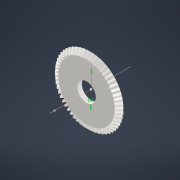
# Autodesk Inventor part: Bevel Gear1
Saved by Autodesk Inventor 2022 (Build 260153000, 153)
## iProperties
CustomPartVersion: 1
Created: 2021-09-10
Part Number: Bevel Gear1
Material: Steel, Mild
Document SubType Name: Modeling
Designer: Andres
Categories: <?xml version="1.0" encoding="UTF-16"?> <MemberInstance><Categories><FamilyTemplate><FamilyTemplateParameter ValueType="xs:double" Id="1" ObjectReferenceKey="da_z" ObjectType="kUserParameterObject"/><FamilyTemplateParameter ValueType="xs:double" Id="2" ObjectReferenceKey="da_b" ObjectType="kUserParameterObject"/><FamilyTemplateParameter ValueType="xs:double" Id="3" ObjectReferenceKey="da_beta" ObjectType="kUserParameterObject"/><FamilyTemplateParameter ValueType="xs:double" Id="4" ObjectReferenceKey="da_dae" ObjectType="kUserParameterObject"/><FamilyTemplateParameter ValueType="xs:double" Id="5" ObjectReferenceKey="da_ve" ObjectType="kUserParameterObject"/><FamilyTemplateParameter ValueType="xs:double" Id="6" ObjectReferenceKey="da_omega" ObjectType="kUserParameterObject"/><FamilyTemplateParameter ValueType="xs:string" Id="7" ObjectReferenceKey="EAIAABAAAAAAHwAAAAAAAIAAAAAAAAAA" ObjectType="83914240" SubObjectId="SurfaceGeometry"/></FamilyTemplate><ParamToTemplateMap><ParamToTemplate CategoryParameter="//CategoryParameter[@InternalName='046C89C9-8512-4d59-83FE-43B91F4F132A']" TemplateParameter="1"/><ParamToTemplate CategoryParameter="//CategoryParameter[@InternalName='2552DF32-E462-4b46-AEBF-C6C7768E72AC']" TemplateParameter="2"/><ParamToTemplate CategoryParameter="//CategoryParameter[@InternalName='C9EE641D-15FC-4fae-A226-E94C4372FDD7']" TemplateParameter="3"/><ParamToTemplate><ParamToTemplate CategoryParameter="//CategoryParameter[@InternalName='00B6519A-459B-49c7-AD84-2E56D39A5744']" ConstantValue="0.000000"/></ParamToTemplate><ParamToTemplate><ParamToTemplate CategoryParameter="//CategoryParameter[@InternalName='04B31F0E-C7A6-4894-AA32-9629BEFACF47']" ConstantValue="1.000000"/></ParamToTemplate><ParamToTemplate><ParamToTemplate CategoryParameter="//CategoryParameter[@InternalName='43CBEC2E-7847-49e7-A936-2F7889FCB2D9']" ConstantValue="0.200000"/></ParamToTemplate><ParamToTemplate><ParamToTemplate CategoryParameter="//CategoryParameter[@InternalName='B1EFC894-105D-4ebd-86BF-FA20ED196853']" ConstantValue="0.300000"/></ParamToTemplate><ParamToTemplate><ParamToTemplate CategoryParameter="//CategoryParameter[@InternalName='51175063-3D10-4879-93E8-6246FE8B403D']" ConstantValue="2060000000.000000"/></ParamToTemplate><ParamToTemplate><ParamToTemplate CategoryParameter="//CategoryParameter[@InternalName='A3A52E27-4454-46a9-B0BD-C932399B70AF']" ConstantValue="0.300000"/></ParamToTemplate><ParamToTemplate CategoryParameter="//CategoryParameter[@InternalName='2A200944-5A8C-41ca-B96E-8520D2E510F1']" TemplateParameter="4"/><ParamToTemplate><ParamToTemplate CategoryParameter="//CategoryParameter[@InternalName='1A637F62-92C8-44bc-B81F-10802510B579']" ConstantValue="9.677909"/></ParamToTemplate><ParamToTemplate CategoryParameter="//CategoryParameter[@InternalName='B52DD4BE-6863-48fb-BF58-89EF6F9EC65C']" TemplateParameter="5"/><ParamToTemplate><ParamToTemplate CategoryParameter="//CategoryParameter[@InternalName='3956BFF2-84D2-457d-93C2-9B0613DEBA67']" ConstantValue="4.854017"/></ParamToTemplate><ParamToTemplate CategoryParameter="//CategoryParameter[@InternalName='739CFA02-461B-4bf8-8049-181FCAD8B28F']" TemplateParameter="6"/><ParamToTemplate><ParamToTemplate CategoryParameter="//CategoryParameter[@InternalName='A27E999F-E2CE-4481-8A2A-EBF499C4C3C5']" ConstantValue="0.000000"/></ParamToTemplate><ParamToTemplate><ParamToTemplate CategoryParameter="//CategoryParameter[@InternalName='9E1B4470-B2D3-4ff1-B813-535BB4CDF51A']" ConstantValue="3520000.000000"/></ParamToTemplate><ParamToTemplate><ParamToTemplate CategoryParameter="//CategoryParameter[@InternalName='F8452263-BFF6-458c-9FB1-07C4B99E95CD']" ConstantValue="11400000.000000"/></ParamToTemplate><ParamToTemplate><ParamToTemplate CategoryParameter="//CategoryParameter[@InternalName='3E3BB259-FD49-497f-8171-6EBC954A3479']" ConstantValue="2.000000"/></ParamToTemplate><ParamToTemplate CategoryParameter="//CategoryParameter[@InternalName='27C3BAF2-7550-4e4b-AE2C-0DB134B7D9B7']" TemplateParameter="7"/></ParamToTemplateMap><Category DisplayName="Gear" InternalName="DC85795E-93AB-48d5-8EEE-5A27447B64BD" Mnemonic="Gear"><CategoryParameter DisplayName="z" InternalName="046C89C9-8512-4d59-83FE-43B91F4F132A" Mnemonic="z"/><CategoryParameter DisplayName="b" InternalName="2552DF32-E462-4b46-AEBF-C6C7768E72AC" Mnemonic="b"/><CategoryParameter DisplayName="||b|" InternalName="C9EE641D-15FC-4fae-A226-E94C4372FDD7" Mnemonic="beta"/><CategoryParameter DisplayName="x" InternalName="00B6519A-459B-49c7-AD84-2E56D39A5744" Mnemonic="x"/><CategoryParameter DisplayName="a*" InternalName="04B31F0E-C7A6-4894-AA32-9629BEFACF47" Mnemonic="a"/><CategoryParameter DisplayName="c*" InternalName="43CBEC2E-7847-49e7-A936-2F7889FCB2D9" Mnemonic="c"/><CategoryParameter DisplayName="r|.f|*" InternalName="B1EFC894-105D-4ebd-86BF-FA20ED196853" Mnemonic="rf"/><CategoryParameter DisplayName="E" InternalName="51175063-3D10-4879-93E8-6246FE8B403D" Mnemonic="E"/><CategoryParameter DisplayName="||m|" InternalName="A3A52E27-4454-46a9-B0BD-C932399B70AF" Mnemonic="mi"/><Category DisplayName="BevelGear" InternalName="0C98F69A-0C2B-4791-B2FE-7691BB227E77" Mnemonic="BevelGear"><CategoryParameter DisplayName="d|.ae|" InternalName="2A200944-5A8C-41ca-B96E-8520D2E510F1" Mnemonic="dae"/><CategoryParameter DisplayName="d|.ai|" InternalName="1A637F62-92C8-44bc-B81F-10802510B579" Mnemonic="dai"/><CategoryParameter DisplayName="A|.e|" InternalName="B52DD4BE-6863-48fb-BF58-89EF6F9EC65C" Mnemonic="ve"/><CategoryParameter DisplayName="A|.i|" InternalName="3956BFF2-84D2-457d-93C2-9B0613DEBA67" Mnemonic="vi"/><CategoryParameter DisplayName="||S|" InternalName="739CFA02-461B-4bf8-8049-181FCAD8B28F" Mnemonic="omega"/><CategoryParameter DisplayName="x|.t|" InternalName="A27E999F-E2CE-4481-8A2A-EBF499C4C3C5" Mnemonic="xt"/><CategoryParameter DisplayName="||s||.Flim|" InternalName="9E1B4470-B2D3-4ff1-B813-535BB4CDF51A" Mnemonic="sFlim"/><CategoryParameter DisplayName="||s||.Hlim|" InternalName="F8452263-BFF6-458c-9FB1-07C4B99E95CD" Mnemonic="sHlim"/><CategoryParameter DisplayName="type" InternalName="3E3BB259-FD49-497f-8171-6EBC954A3479" Mnemonic="type"/><CategoryParameter DisplayName="PitchDiameter" InternalName="27C3BAF2-7550-4e4b-AE2C-0DB134B7D9B7" Mnemonic="IDS_PITCHDIAM"/></Category></Category></Categories></MemberInstance>
Mass: 60.9118 g
Surface Area: 34.3074 cm^2
Volume: 7.7496 cm^3
Density: 7.86 g/cm^3
Appearance: Steel
Author: Andres
Autodesk Inventor part; units mm, degrees
ref_plane "Mesh Plane2" through (0, 0, 0) normal (0.9983082, 0.0581448, 0) x (0, 0, 1)
sketch "Teeth Body Sketch" plane through (0, 0, 0) normal (1, 0, 0) x (0, 1, 0)
  line L0 (0, 0) -> (52.2577, -58.6506) construction
  line L1 (52.2577, -58.6506) -> (55.4519, -55.6245)
  line L2 (55.4519, -55.6245) -> (0, 0) construction
  line L3 (54, -57) -> (0, 0) construction
  line L4 (45.6022, -51.1808) -> (48.3895, -48.5402)
  line L5 (52.2577, -58.6506) -> (45.6022, -51.1808)
  line L6 (55.4519, -55.6245) -> (48.3895, -48.5402)
  line L7 (0, -70.5507) -> (0, 11.7584) projected
  line L8 (0, -57) -> (55.4519, -57) construction
  dimension "d0" = 108
  dimension "d1" = 104.5154
  dimension "d2" = 110.9038
  dimension "d3" = 10
  dimension "d4" = 55.6245
  constraints: 16 end point, 4 point on line, 3 perpendicular, 2 collinear, 1 horizontal alignment, 1 vertical alignment
  measures "d0" diameter of L3.start L7
  measures "d1" diameter of L0.end L7
  measures "d2" diameter of L1.end L7
  measures "d3" distance between parallel lines of L1 L4
  measures "d4" vertical distance of L1.end L0.start
revolve "Teeth Body" add sketch "Teeth Body Sketch" angle 360 about axis through (0, 0, 0) along (0, 0, 1)
ref_plane "Tooth Plane" through (0, 54, -57) normal (0, -0.6877446, 0.7259527) x (1, 0, 0)
sketch "Start Sketch" plane through (0, 54, -57) normal (0, -0.6877446, 0.7259527) x (1, 0, 0)
  line L0 (0, -116.14) -> (0, 23.2448) projected
  arc A0 (-0.6771, -2.928) -> (-3.0931, 3.2584) centre (-26.0317, -9.265) ccw
  arc A1 (3.0931, 3.2584) -> (0.6771, -2.928) centre (26.0317, -9.265) ccw
  line L1 (-0.6771, -2.928) -> (0.6771, -2.928)
  arc A2 (3.0931, 3.2584) -> (-3.0931, 3.2584) centre (0, -74.385) ccw
  dimension "d7" = 26.1346
  dimension "d8" = 26.0317
  dimension "d9" = 65.1201
  dimension "d57" = 77.705
  dimension "d58" = 71.457
  constraints: 6 point on circle, 3 centre point, 3 symmetric about line, 2 end point, 1 coincident, 1 perpendicular, 1 other
  measures "d7" radius of A0
  measures "d8" horizontal distance of point (0, -74.385) A0.centre
  measures "d9" vertical distance of point (0, -74.385) A0.centre
  measures "d57" radius of A2
  measures "d58" distance from line of A2.centre L1
sketch "End Sketch" plane through (0, 46.9712, -49.5808) normal (0, -0.6877446, 0.7259527) x (1, 0, 0)
  line L0 (0, -102.2904) -> (0, 20.4729) projected
  arc A0 (-0.589, -2.5469) -> (-2.6905, 2.8343) centre (-22.6434, -8.059) ccw
  arc A1 (2.6905, 2.8343) -> (0.589, -2.5469) centre (22.6434, -8.059) ccw
  line L1 (-0.589, -2.5469) -> (0.589, -2.5469)
  arc A2 (2.6905, 2.8343) -> (-2.6905, 2.8343) centre (0, -64.7029) ccw
  dimension "d12" = 22.7328
  dimension "d15" = 22.6434
  dimension "d16" = 56.6439
  dimension "d59" = 67.5908
  dimension "d60" = 62.156
  constraints: 6 point on circle, 3 centre point, 3 symmetric about line, 2 end point, 1 coincident, 1 other
  measures "d12" radius of A0
  measures "d15" horizontal distance of A0.centre point (0, -64.703)
  measures "d16" vertical distance of A0.centre point (0, -64.703)
  measures "d59" radius of A2
  measures "d60" distance from line of A2.centre L1
loft "Loft" cut profiles "Start Sketch", "End Sketch"
pattern_circular "Circular Pattern" count 54 over 360 about axis through (0, 0, 0) along (0, 0, 1) of "Loft"
ref_plane "End Plane" through (0, 46.9712, -49.5808) normal (0, -0.6877446, 0.7259527) x (1, 0, 0)
sketch3d "3D Sketch Right"
ref_plane "End Plane Right" through (-3.2641, 46.8577, -49.5808) normal (0.0477919, -0.6860821, 0.7259527) x (0.9975826, 0.0694908, 0)
sketch "End Sketch Right" plane through (-3.2641, 46.8577, -49.5808) normal (0.0477919, -0.6860821, 0.7259527) x (0.9975826, 0.0694908, 0)
  arc A0 (-0.589, -2.5469) -> (-2.6905, 2.8343) centre (-22.6434, -8.059) ccw
  line L0 (0, -106.3985) -> (0, 24.581) projected
  arc A1 (2.6905, 2.8343) -> (0.589, -2.5469) centre (22.6434, -8.059) ccw
  line L1 (-0.589, -2.5469) -> (0.589, -2.5469)
  arc A2 (2.6905, 2.8343) -> (-2.6905, 2.8343) centre (0, -64.7029) ccw
  dimension "d70" = 22.6434
  dimension "d71" = 56.6439
  dimension "d72" = 22.7328
  dimension "d73" = 62.156
  dimension "d74" = 67.5908
  constraints: 6 point on circle, 3 centre point, 3 symmetric about line, 2 end point, 1 coincident, 1 perpendicular, 1 other
  measures "d70" horizontal distance of A2.centre A0.centre
  measures "d71" vertical distance of point (0, -64.703) A0.centre
  measures "d72" radius of A0
  measures "d73" distance from line of point (0, -64.703) L1
  measures "d74" radius of A2
feature "Loft Right" [suppressed]
pattern_circular "Circular Pattern Right" [suppressed]
sketch3d "3D Sketch Left"
ref_plane "End Plane Left" through (3.2651, 46.8577, -49.5812) normal (-0.047807, -0.6860782, 0.7259554) x (0.997581, -0.069513, 0)
sketch "End Sketch Left" plane through (3.2651, 46.8577, -49.5812) normal (-0.047807, -0.6860782, 0.7259554) x (0.997581, -0.069513, 0)
  line L0 (0, -110.4238) -> (0, 28.6078) projected
  arc A0 (-0.589, -2.5466) -> (-2.6905, 2.8346) centre (-22.6434, -8.0587) ccw
  arc A1 (2.6905, 2.8346) -> (0.589, -2.5466) centre (22.6434, -8.0587) ccw
  line L1 (-0.589, -2.5466) -> (0.589, -2.5466)
  ellipse E0 centre (0, -33.3831) end of major axis (48.3895, -33.3831) minor radius 35.1286 projected
  arc A2 (2.6905, 2.8346) -> (-2.6905, 2.8346) centre (0, -64.7026) ccw
  dimension "d56" = 35.1287
  dimension "d30" = 22.7328
  dimension "d31" = 22.6434
  dimension "d32" = 56.6439
  dimension "d61" = 67.5908
  dimension "d62" = 62.156
  constraints: 6 point on circle, 3 centre point, 3 symmetric about line, 2 end point, 1 coincident, 2 other
  measures "d30" radius of A0
  measures "d31" horizontal distance of point (0, -64.703) A0.centre
  measures "d32" vertical distance of A0.centre point (0, -64.703)
  measures "d61" radius of A2
  measures "d62" distance from line of point (0, -64.703) L1
feature "Loft Left" [suppressed]
pattern_circular "Circular Pattern Left" [suppressed]
sketch "Body Sketch" plane through (0, 0, 0) normal (1, 0, 0) x (0, 1, 0)
  line L0 (0, -60.1642) -> (0, -50.5602) projected
  line L1 (52.2577, -58.6506) -> (45.6022, -51.1808) projected
  line L2 (45.6022, -51.1808) -> (0, -51.1808)
  line L3 (52.2577, -58.6506) -> (0, -58.6506)
  constraints: 4 end point, 2 perpendicular, 2 point on line
revolve "Fix Body" add sketch "Body Sketch" angle 360 about axis through (0, 0, 0) along (0, 0, 1)
sketch "Sketch6" plane through (0, 0, 0) normal (1, 0, 0) x (0, 1, 0)
  line L0 (54, -57) -> (0, 0) projected
  line L1 (0, -68.4) -> (0, 11.4) projected
surface revolve "Pitch Diameter" sketch "Sketch6" angle 360 about axis through (0, 0, 0) along (0, 0, 1) shown no curves L0
sketch "Sketch8" plane through (0, 0, -58.6506) normal (0, 0, -1) x (-0.9986295, 0.052336, 0)
  circle A0 centre (0, 0) radius 15
  dimension "d99" = 30
  constraints: 1 centre point, 1 coincident
  measures "d99" diameter of A0
extrude "Extrusion1" cut sketch "Sketch8" against normal through all
sketch "Sketch10" plane through (0, 0, -58.6506) normal (0, 0, 1) x (1, 0, 0)
  circle A0 centre (-6.3642, 21.5812) radius 1.2295 projected
  circle A1 centre (-21.872, 5.279) radius 1.2295 projected
  circle A2 centre (-15.5077, -16.3022) radius 1.2295 projected
  circle A3 centre (6.3642, -21.5812) radius 1.2295 projected
  circle A4 centre (21.872, -5.279) radius 1.2295 projected
  circle A5 centre (15.5077, 16.3022) radius 1.2295 projected
  circle A6 centre (0, 0) radius 30 projected
  circle A7 centre (0, 0) radius 8 projected
  point P0 (0, 0)
hole "Hole1" at (15.5077, 16.3022, -58.6506) at (21.872, -5.279, -58.6506) at (6.3642, -21.5812, -58.6506) at (-15.5077, -16.3022, -58.6506) at (-21.872, 5.279, -58.6506) at (-6.3642, 21.5812, -58.6506) direction (0, 0, 1) diameter 3.4 depth 7.4697 counterbore diameter 6 counterbore depth 2.6 clearance for "Hex Head Cap Screw ISO 24017" size "M3" standard "ISO"
equation "\"d0\" = da_de"
equation "\"d1\" = da_dfe"
equation "\"d2\" = da_dae"
equation "\"d3\" = da_b"
equation "\"d4\" = da_ve"
equation "\"d7\" = fd_rr"
equation "\"d8\" = fd_x"
equation "\"d9\" = fd_y"
equation "\"d57\" = 0.5 * fd_dva + 0.3 * da_he"
equation "\"d58\" = 0.5 * fd_dva - 1.12 * da_he"
equation "\"da_teethtype\" = 0"
equation "\"da_b\" = 10"
equation "\"da_de\" = 108"
equation "\"da_dae\" = 110.90381"
equation "\"da_dfe\" = 104.51543"
equation "\"da_le\" = 78.51751"
equation "\"da_omega\" = 90deg"
equation "\"da_beta\" = 0"
equation "\"da_delta\" = 43.451842deg"
equation "\"da_alpha\" = 20deg"
equation "\"da_he\" = 4.4"
equation "\"da_ve\" = 55.62451"
equation "\"da_zv\" = 74.385013"
equation "\"fd_loft\" = da_b + 0.05 * da_he"
equation "\"fd_x\" = fd_x1 + fd_x2"
equation "\"fd_y\" = fd_y1 - fd_y2"
equation "\"fd_dd\" = fd_dva - 0.8 * da_he"
equation "\"da_dvw\" = 148.77003"
equation "\"d11\" = fd_loft"
equation "\"da_dm\" = 101.12255"
equation "\"da_x\" = 0"
equation "\"da_m\" = 2"
equation "\"d50\" = da_omega"
equation "\"fd_rr\" = 26.134569"
equation "\"fd_dva\" = 152.770026"
equation "\"fd_x1\" = 1.588129"
equation "\"fd_x2\" = 24.443612"
equation "\"fd_y1\" = 74.368058"
equation "\"fd_y2\" = 9.248"
body "Solid1"
body "Srf1"
